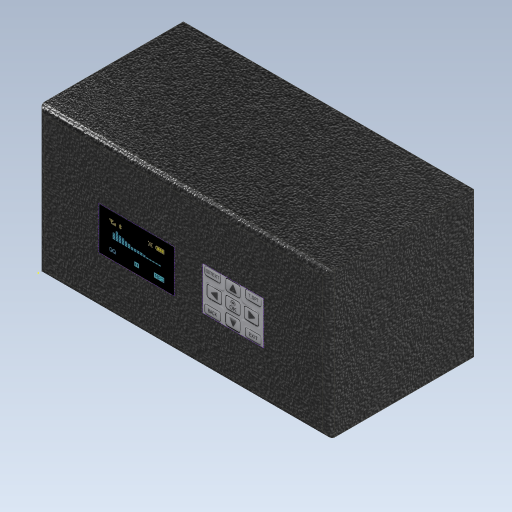
# Autodesk Inventor part: caja
Saved by Autodesk Inventor 2023 (Build 270158000, 158)
## iProperties
Created: 2023-03-08
Part Number: caja
Material: Steel, Wrought
Document SubType Name: Modeling
Designer: santi
Density: 7.85 g/cm^3
Appearance: Steel
Author: santi
Autodesk Inventor part; units mm, degrees
ref_plane "YZ Plane" through (0, 0, 0) normal (1, 0, 0) x (0, 1, 0)
ref_plane "XZ Plane" through (0, 0, 0) normal (0, 1, 0) x (-1, 0, 0)
ref_plane "XY Plane" through (0, 0, 0) normal (0, 0, 1) x (1, 0, 0)
sketch "Sketch1" plane through (0, 0, 0) normal (0, 0, 1) x (1, 0, 0)
  point P0 (0, 0)
sketch "Sketch2" plane through (0, 0, 0) normal (0, 0, 1) x (1, 0, 0)
  line L0 (0, 0) -> (100, 0)
  line L1 (100, 0) -> (100, 50)
  line L2 (100, 50) -> (0, 50)
  line L3 (0, 50) -> (0, 0)
  dimension "d0" = 100
  dimension "d1" = 50
  constraints: 8 end point, 2 parallel, 1 horizontal, 1 perpendicular
  measures "d0" distance of L2.end L1.end
  measures "d1" distance of L1.end L0.end
extrude "Extrusion1" add sketch "Sketch2" along normal blind 50
sketch "Sketch3" plane through (0, 0, 50) normal (0, 0, 1) x (1, 0, 0)
  line L0 (20.8812, 31.3356) -> (46.8519, 31.3356) construction
  line L1 (46.8519, 31.3356) -> (46.8519, 16.5581) construction
  line L2 (46.8519, 16.5581) -> (20.8812, 16.5581) construction
  line L3 (20.8812, 16.5581) -> (20.8812, 31.3356) construction
  line L4 (56.6371, 31.214) -> (77.5699, 31.214) construction
  line L5 (77.5699, 31.214) -> (77.5699, 16.4712) construction
  line L6 (77.5699, 16.4712) -> (56.6371, 16.4712) construction
  line L7 (56.6371, 16.4712) -> (56.6371, 31.214) construction
  point P0 (0, 0)
  constraints: 4 other
fillet "Fillet2" radius 2 4 edges at (0, 25, 50) (50, 50, 50) (50, 0, 50) (100, 25, 50)
body "Solid1"
